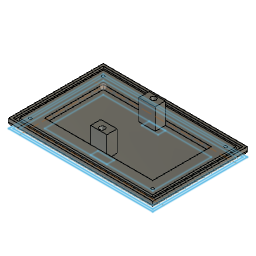
Rad Box Top v3 (Autodesk Fusion 360 design; units mm, degrees)
Autodesk Fusion 360 part; units mm, degrees
note: some values were not read from the file. Chosen so that the rebuilt part matches the saved one: that a step has no effect.
sketch "BottomofboxBox" plane through (0, 0, 0) normal (0, 0, 1) x (1, 0, 0)
  line L0 (-325, 75) -> (-165, 75)
  line L1 (-165, 75) -> (-165, -30)
  line L2 (-165, -30) -> (-325, -30)
  line L3 (-325, -30) -> (-325, 75)
  line L4 (-325, 63) -> (-313, 63) construction
  line L5 (-313, 63) -> (-165, 63) construction
  line L6 (-313, 63) -> (-313, -30) construction
  line L7 (-325, -18) -> (-165, -18) construction
  line L8 (-322.5, -27.5) -> (-167.5, -27.5)
  line L9 (-167.5, -27.5) -> (-167.5, 72.5)
  line L10 (-167.5, 72.5) -> (-322.5, 72.5)
  line L11 (-322.5, 72.5) -> (-322.5, -27.5)
  line L12 (-318.86, -23.86) -> (-171.14, -23.86)
  line L13 (-171.14, -23.86) -> (-171.14, 68.86)
  line L14 (-171.14, 68.86) -> (-318.86, 68.86)
  line L15 (-318.86, 68.86) -> (-318.86, -23.86)
  line L16 (-305, -10) -> (-185, -10)
  line L17 (-185, -10) -> (-185, 55)
  line L18 (-185, 55) -> (-305, 55)
  line L19 (-305, 55) -> (-305, -10)
  line L20 (-254, 55) -> (-236, 55)
  line L21 (-236, 55) -> (-236, 47)
  line L22 (-236, 47) -> (-254, 47)
  line L23 (-254, 47) -> (-254, 55)
  line L24 (-236, -2) -> (-236, -10)
  line L25 (-254, -2) -> (-236, -2)
  line L26 (-236, -10) -> (-254, -10)
  line L27 (-254, -10) -> (-254, -2)
  dimension "d1" = 160
  dimension "d2" = 105
  dimension "d4" = 12
  dimension "d5" = 12
  dimension "d6" = 12
  dimension "d58" = 2.5
  dimension "d59" = 2.5
  dimension "d60" = 2.5
  dimension "d61" = 12
  dimension "d62" = 6.14
  dimension "d63" = 6.14
  dimension "d64" = 6.14
  dimension "d65" = 6.14
  dimension "d66" = 2.5
  dimension "d69" = 20
  dimension "d70" = 20
  dimension "d71" = 20
  dimension "d72" = 20
  dimension "d91" = 18
  dimension "d92" = 51
  dimension "d93" = 8
  dimension "d94" = 18
  dimension "d95" = 8
  constraint horizontal L0
  constraint vertical L1
  constraint horizontal L2
  constraint vertical L3
  constraint coincident L3 L4.start
  constraint perpendicular L3 L4
  constraint coincident L1 L5.end
  constraint perpendicular L1 L5
  constraint coincident L2 L6.end
  constraint perpendicular L2 L6
  constraint coincident L3 L7.start
  constraint coincident L1 L7.end
  constraint perpendicular L1 L7
  constraint horizontal L8
  constraint vertical L9
  constraint horizontal L10
  constraint vertical L11
  constraint horizontal L12
  constraint vertical L13
  constraint horizontal L14
  constraint vertical L15
  constraint horizontal L16
  constraint vertical L17
  constraint horizontal L18
  constraint vertical L19
  constraint horizontal L20
  constraint vertical L21
  constraint horizontal L22
  constraint vertical L23
  constraint coincident L18 L20.start
  constraint horizontal L25
  constraint vertical L24
  constraint horizontal L26
  constraint vertical L27
  measures "d1" distance of L0.start L0.end
  measures "d2" distance of L0.start L2.end
  measures "d4" distance of L3 L4.end
  measures "d5" distance of L0 L4.end
  measures "d6" distance of L2.end L7.start
  measures "d58" distance of L2 L8.start
  measures "d59" distance of L3 L8.start
  measures "d60" distance of L0 L10.end
  measures "d61" distance of L0 L4.end
  measures "d62" distance of L3 L12.start
  measures "d63" distance of L2 L12.end
  measures "d64" distance of L0 L14.end
  measures "d65" distance of L1 L13.end
  measures "d66" distance of L1 L9.end
  measures "d69" distance of L3 L16.start
  measures "d70" distance of L0 L18.end
  measures "d71" distance of L1 L16.end
  measures "d72" distance of L2 L16.end
  measures "d91" distance of L21.end L22.end
  measures "d92" distance of L18.end L20.start
  measures "d93" distance of L20.end L21.end
  measures "d94" distance of L24.end L26.end
  measures "d95" distance of L24.end L24.start
extrude "Extrude22" add sketch "BottomofboxBox" along normal blind 28 contours L16 L24 L25 L26 L27 makes body 1
extrude "Extrude19" add sketch "BottomofboxBox" along normal blind 26 separate body contours L18 L20 L21 L22 L23 makes body 2
extrude "Extrude16" add sketch "BottomofboxBox" along normal blind 2 separate body contours L8 L9 L10 L11 makes body 3
extrude "Extrude13" add sketch "BottomofboxBox" along normal blind 1.1 separate body contours L8 L9 L10 L11 makes body 4
extrude "Extrude10" add sketch "BottomofboxBox" against normal blind 5 separate body contours L16 L17 L18 L19 L21 L22 L23 L24 L25 L27 | L16 L24 L25 L26 L27 | L18 L20 L21 L22 L23 makes body 5
extrude "Extrude6" add sketch "BottomofboxBox" along normal blind 8 separate body contours L0 L1 L2 L3 | L8 L9 L10 L11 | L12 L13 L14 L15 | L16 L17 L18 L19 L21 L22 L23 L24 L25 L27 | L16 L24 L25 L26 L27 | L18 L20 L21 L22 L23 makes body 6
sketch "TopOf Box" plane through (0, 0, 8) normal (0, 0, 1) x (-1, 0, 0)
  line L0 (325, 30) -> (165, 30)
  line L1 (165, 30) -> (165, -75)
  line L2 (165, -75) -> (325, -75)
  line L3 (325, -75) -> (325, 30)
  line L4 (325, 18) -> (165, 18) construction
  line L5 (313, -75) -> (313, 30) construction
  line L6 (325, -63) -> (165, -63) construction
  line L7 (177, -75) -> (177, 30) construction
  circle A0 centre (313, -63) radius 3.5 construction
  circle A1 centre (313, -63) radius 1.5 construction
  circle A2 centre (313, -63) radius 3.5 construction
  circle A3 centre (313, -63) radius 1.5
  circle A4 centre (313, -63) radius 3.5
  circle A5 centre (313, 18) radius 3.5
  circle A6 centre (313, 18) radius 3.5 construction
  circle A7 centre (313, 18) radius 1.5 construction
  circle A8 centre (313, 18) radius 3.5 construction
  circle A9 centre (313, 18) radius 1.5
  circle A10 centre (177, -63) radius 3.5
  circle A11 centre (177, -63) radius 3.5 construction
  circle A12 centre (177, -63) radius 1.5 construction
  circle A13 centre (177, -63) radius 3.5 construction
  circle A14 centre (177, -63) radius 1.5
  circle A15 centre (177, 18) radius 3.5
  circle A16 centre (177, 18) radius 3.5 construction
  circle A17 centre (177, 18) radius 1.5 construction
  circle A18 centre (177, 18) radius 3.5 construction
  circle A19 centre (177, 18) radius 1.5
  point P0 (313, -63)
  point P1 (313, 18)
  point P2 (177, -63)
  point P3 (177, 18)
  dimension "d28" = 12
  dimension "d29" = 12
  dimension "d30" = 12
  dimension "d31" = 12
  dimension "d32" = 7
  dimension "d33" = 3
  dimension "d34" = 7
  dimension "d35" = 3
  dimension "d36" = 7
  dimension "d37" = 7
  dimension "d38" = 3
  dimension "d39" = 7
  dimension "d40" = 3
  dimension "d41" = 7
  dimension "d42" = 7
  dimension "d43" = 3
  dimension "d44" = 7
  dimension "d45" = 3
  dimension "d46" = 7
  dimension "d47" = 7
  dimension "d48" = 3
  dimension "d49" = 7
  dimension "d50" = 3
  dimension "d51" = 7
  constraint coincident L3 L4.start
  constraint perpendicular L3 L4
  constraint coincident L2 L5.start
  constraint coincident L0 L5.end
  constraint perpendicular L0 L5
  constraint coincident L3 L6.start
  constraint coincident L1 L6.end
  constraint perpendicular L1 L6
  constraint coincident L2 L7.start
  constraint coincident L0 L7.end
  constraint perpendicular L0 L7
  constraint coincident L5 P0
  constraint coincident L6 P0
  constraint concentric A0 A1
  constraint concentric A2 A3
  constraint concentric A6 A7
  constraint concentric A8 A9
  constraint concentric A11 A12
  constraint concentric A13 A14
  constraint concentric A16 A17
  constraint concentric A18 A19
  measures "d28" distance of L0.start L4.start
  measures "d29" distance of L0.start L5.end
  measures "d30" distance of L1.end L7.start
  measures "d31" distance of L1.end L6.end
  measures "d32" diameter of A0
  measures "d33" diameter of A1
  measures "d34" diameter of A2
  measures "d35" diameter of A3
  measures "d36" diameter of A4
  measures "d37" diameter of A6
  measures "d38" diameter of A7
  measures "d39" diameter of A8
  measures "d40" diameter of A9
  measures "d41" diameter of A5
  measures "d42" diameter of A11
  measures "d43" diameter of A12
  measures "d44" diameter of A13
  measures "d45" diameter of A14
  measures "d46" diameter of A10
  measures "d47" diameter of A16
  measures "d48" diameter of A17
  measures "d49" diameter of A18
  measures "d50" diameter of A19
  measures "d51" diameter of A15
extrude "Extrude8" cut sketch "TopOf Box" against normal blind 10 contours A3 | A9 | A14 | A19 bodies 6
extrude "Extrude7" cut sketch "TopOf Box" against normal blind 4 contours A4 | A5 | A10 | A15 bodies 6
fillet "Fillet1" radius 4 4 edges at (-325, 22.5, 8) (-245, -30, 8) (-165, 22.5, 8) (-245, 75, 8) on bodies 6
extrude "Extrude9" add sketch "BottomofboxBox" along normal blind 1.5 contours L8 L9 L10 L11 bodies 6 4
extrude "Extrude11" cut 1 faces at (-265, 33.3333, -5) along direction (0, 0, 1) blind 5 on bodies 5 bodies 5
extrude "Extrude12" cut sketch "BottomofboxBox" along normal blind 5 contours L16 L17 L18 L19 L21 L22 L23 L24 L25 L27 | L16 L24 L25 L26 L27 | L18 L20 L21 L22 L23 bodies 6
extrude "Extrude15" [no effect]
extrude "Extrude17" cut sketch "BottomofboxBox" along normal blind 2.25 contours L8 L9 L10 L11 bodies 3 6
move_body "Move1" bodies 6 to x (1, 0, 0) y (0, -1, 0) z (0, 0, -1) at (0, 45, 10)
combine "Combine2" [no effect]
extrude "Extrude20" cut 1 faces at (-248, 52.3333, 0) along direction (0, 0, 1) blind 2 on bodies 2 bodies 2
extrude "Extrude21" add 1 faces at (-248, 52.3333, 26) along direction (0, 0, 1) blind 2 on bodies 2 bodies 2
extrude "Extrude23" add sketch "BottomofboxBox" against normal blind 2 contours L16 L24 L25 L26 L27 bodies 1
extrude "Extrude24" cut 1 faces at (-248, -4.6667, -2) along direction (0, 0, 1) blind 2 on bodies 1 bodies 1
extrude "Extrude25" cut sketch "BottomofboxBox" along normal blind 2 contours L16 L24 L25 L26 L27 bodies 1
sketch "Sketch3" plane through (0, 0, 28) normal (0, 0, 1) x (-1, 0, 0)
  line L0 (254, -47) -> (236, -47)
  line L1 (236, -47) -> (236, -55)
  line L2 (236, -55) -> (254, -55)
  line L3 (254, -55) -> (254, -47)
  circle A0 centre (245, -51) radius 2.9
  dimension "d113" = 5.8
  measures "d113" diameter of A0
extrude "Extrude26" cut sketch "Sketch3" against normal blind 6 contours A0 bodies 2
sketch "Sketch4" plane through (0, 0, 28) normal (0, 0, 1) x (-1, 0, 0)
  line L0 (254, 10) -> (236, 10)
  line L1 (236, 10) -> (236, 2)
  line L2 (236, 2) -> (254, 2)
  line L3 (254, 2) -> (254, 10)
  circle A0 centre (245, 6.0084) radius 2.9
  dimension "d116" = 5.8
  measures "d116" diameter of A0
extrude "Extrude27" cut sketch "Sketch4" against normal blind 6 contours A0 bodies 1
extrude "Extrude28" add 1 faces at (-238.0333, 51, 28) along direction (0, 0, 1) blind 1.5 on bodies 2 bodies 2
extrude "Extrude29" add 1 faces at (-251.9667, -6.0028, 28) along direction (0, 0, 1) blind 1.5 on bodies 1 bodies 1
extrude "Extrude30" add 1 faces at (-242, 47, 11.1667) along direction (0, -1, 0) blind 3.3 on bodies 2 bodies 2 1 6
extrude "Extrude31" add 1 faces at (-248, -2, 11.1667) along direction (0, 1, 0) blind 3.3 on bodies 1 bodies 1 2
extrude "Extrude32" cut 1 faces at (-251.9559, -4.7587, 29.5) along direction (0, 0, -1) blind 1 on bodies 1 bodies 1
extrude "Extrude33" cut 1 faces at (-238.0441, 49.7559, 29.5) along direction (0, 0, -1) blind 1 on bodies 1 bodies 1
equation "insidetophole = 3 mm"
equation "d33 = insidetophole"
equation "d35 = insidetophole"
equation "d38 = insidetophole"
equation "d40 = insidetophole"
equation "d43 = insidetophole"
equation "d45 = insidetophole"
equation "d48 = insidetophole"
equation "d50 = insidetophole"
equation "BIHole = 5.8 mm"
equation "d113 = BIHole"
equation "d116 = BIHole"
